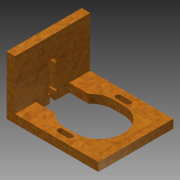
# Autodesk Inventor part: frame_x
Saved by Autodesk Inventor 2014 (Build 180170000, 170)
## iProperties
Created: 2015-01-04
Part Number: frame_x
Material: Generic
Document SubType Name: Modeling
Designer: cruiser
Density: 1 g/cm^3
Appearance: Yellow Pine - Solid Stained Light Low Gloss
Author: cruiser
Autodesk Inventor part; units mm, degrees
ref_plane "YZ Plane" through (0, 0, 0) normal (1, 0, 0) x (0, 1, 0)
ref_plane "XZ Plane" through (0, 0, 0) normal (0, 1, 0) x (-1, 0, 0)
ref_plane "XY Plane" through (0, 0, 0) normal (0, 0, 1) x (1, 0, 0)
sketch "Sketch1" plane through (0, 0, 0) normal (0, 0, 1) x (1, 0, 0)
  circle A0 centre (0, 0) radius 14.5
  circle A1 centre (0, 17.5) radius 1.575
  line L0 (0, 0) -> (14.5, 0)
  circle A2 centre (0, -17.5) radius 1.575
  line L1 (0, 10) -> (-25, 10)
  line L2 (-25, 10) -> (-25, -10)
  line L3 (-25, -10) -> (0, -10)
  line L4 (0, -10) -> (0, 10)
  line L5 (25, -22.5) -> (-25, -22.5)
  line L6 (-25, -22.5) -> (-25, 22.5)
  line L7 (-25, 22.5) -> (25, 22.5)
  line L8 (25, 22.5) -> (25, -22.5)
  line L9 (25, -22.5) -> (-25, 22.5) construction
  line L10 (-25, -22.5) -> (25, 22.5) construction
  dimension "d1" = 29
  dimension "d0" = 3.15
  dimension "d2" = 17.5
  dimension "d3" = 0
  dimension "d4" = 20
  dimension "d5" = 25
  dimension "d6" = 0
  dimension "d7" = 50
  dimension "d8" = 45
  constraints: 22 end point, 4 parallel, 3 horizontal, 2 centre point, 2 midpoint, 2 perpendicular, 1 coincident, 1 horizontal alignment, 1 symmetric about line, 4 other
  measures "d0" diameter of A1
  measures "d2" distance of point (0, 0) A1.centre
  measures "d3" horizontal distance of point (0, 0) A1.centre
  measures "d4" distance of L1.end L2.end
  measures "d5" distance from line of A1.centre L2
  measures "d6" distance from line of L4 point (0, 0)
  measures "d7" distance of L6.end L7.end
  measures "d8" distance of L5.end L6.end
extrude "Extrusion1" add sketch "Sketch1" along normal blind 5.08 contours A0 L1 L6 L7 L8 L5 L3
sketch "Sketch2" plane through (-25, 10, 0) normal (-1, 0, 0) x (0, 0, 1)
  line L0 (0, 0) -> (0, 12.5) projected
  line L1 (0, -32.5) -> (5.08, -32.5)
  line L2 (5.08, -32.5) -> (5.08, 12.5)
  line L3 (5.08, 12.5) -> (0, 12.5)
  line L4 (0, 12.5) -> (0, -32.5)
  line L5 (0, -32.5) -> (5.08, -32.5) projected
  point P0 (0, -10)
  dimension "d11" = 0
  dimension "d12" = 0
  constraints: 8 end point, 2 parallel, 1 horizontal, 1 perpendicular
  measures "d11" distance between parallel lines of L4 L0
  measures "d12" distance between parallel lines of L5 L1
extrude "Extrusion2" add sketch "Sketch2" along normal blind 5.08 separate body
sketch "Sketch3" plane through (-25, -22.5, 5.08) normal (0, 0, 1) x (1, 0, 0)
  line L0 (0, 0) -> (0, 45) projected
  line L1 (0, 45) -> (-5.08, 45) projected
  line L2 (-5.08, 0) -> (-5.08, 45) projected
  line L3 (0, 0) -> (-5.08, 0) projected
  point P0 (25, 22.5)
extrude "Extrusion3" add sketch "Sketch3" along normal blind 30 bodies 2
sketch "Sketch4" plane through (-25, 10, 0) normal (1, 0, 0) x (0, 0, -1)
  line L0 (-35.08, -32.5) -> (-35.08, 12.5) projected
  line L1 (0, 12.5) -> (0, -32.5) projected
  line L2 (-35.08, -10) -> (0, -10)
  arc A0 (-19.58, -8) -> (-22.58, -8) centre (-21.08, -10) ccw
  line L3 (-19.58, -12) -> (-22.58, -12)
  line L4 (-22.58, -12) -> (-22.58, -8)
  line L5 (-22.58, -8) -> (-19.58, -8)
  line L6 (-19.58, -8) -> (-19.58, -12)
  line L7 (-19.58, -12) -> (-22.58, -8) construction
  line L8 (-22.58, -12) -> (-19.58, -8) construction
  line L9 (-5.08, -32.5) -> (-5.08, 12.5) projected
  arc A1 (-18.58, -10) -> (-19.58, -8) centre (-21.08, -10) ccw
  arc A2 (-22.58, -8) -> (-23.58, -10) centre (-21.08, -10) ccw
  arc A3 (-23.58, -10) -> (-22.58, -12) centre (-21.08, -10) ccw
  arc A4 (-22.58, -12) -> (-19.58, -12) centre (-21.08, -10) ccw
  arc A5 (-19.58, -12) -> (-18.58, -10) centre (-21.08, -10) ccw
  line L10 (0, -11.65) -> (-19.58, -11.65)
  line L11 (-19.58, -11.65) -> (-19.58, -8.35)
  line L12 (-19.58, -8.35) -> (0, -8.35)
  line L13 (0, -8.35) -> (0, -11.65)
  line L14 (0, -11.65) -> (-19.58, -8.35) construction
  line L15 (-19.58, -11.65) -> (0, -8.35) construction
  line L16 (-7.5, -12.75) -> (-5, -12.75)
  line L17 (-5, -12.75) -> (-5, -7.25)
  line L18 (-5, -7.25) -> (-7.5, -7.25)
  line L19 (-7.5, -7.25) -> (-7.5, -12.75)
  line L20 (-7.5, -12.75) -> (-5, -7.25) construction
  line L21 (-5, -12.75) -> (-7.5, -7.25) construction
  point P0 (-9.79, -10)
  point P1 (-6.25, -10)
  dimension "d17" = 5
  dimension "d18" = 3
  dimension "d19" = 16
  dimension "d20" = 3.3
  dimension "d21" = 0
  dimension "d22" = 0
  dimension "d23" = 2.5
  dimension "d24" = 5.5
  dimension "d25" = 5
  constraints: 38 end point, 12 point on circle, 7 midpoint, 6 centre point, 6 parallel, 5 point on line, 4 perpendicular, 3 horizontal
  measures "d17" diameter of A0
  measures "d18" distance of L4.end L5.end
  measures "d19" distance from line of L9 A0.centre
  measures "d20" distance of L10.end L11.end
  measures "d21" distance between parallel lines of L1 L13
  measures "d22" distance between parallel lines of L6 L11
  measures "d23" distance of L18.end L17.end
  measures "d24" distance of L17.end L16.end
  measures "d25" distance between parallel lines of L1 L17
extrude "Extrusion4" cut sketch "Sketch4" against normal up to next contours L1 L2 L17 L12 | L1 L10 L17 L2 | L17 L2 L9 L12 | L12 L9 L18 L17 | L17 L10 L9 L2 | L12 L19 L18 L9 | L9 L2 L19 L12 | L17 L16 L9 L10 | L9 L10 L19 L2 | L19 L2 A1 L12 | L9 L16 L19 L10 | L19 L10 A5 L2 | A1 L2 L6 L12 | A5 L10 L6 L2 | L5 A0 | L6 L2 L4 L5 | L6 L3 L4 L2 | A4 L3 bodies 2
sketch "Sketch5" plane through (-25, 10, 0) normal (1, 0, 0) x (0, 0, -1)
  arc A0 (-22.58, -12) -> (-19.58, -12) centre (-21.08, -10) ccw projected
  arc A1 (-19.58, -8) -> (-22.58, -8) centre (-21.08, -10) ccw projected
  line L0 (-13.08, -27.5) -> (-29.08, -27.5)
  line L1 (-29.08, -27.5) -> (-29.08, 7.5)
  line L2 (-29.08, 7.5) -> (-13.08, 7.5)
  line L3 (-13.08, 7.5) -> (-13.08, -27.5)
  line L4 (-13.08, -27.5) -> (-29.08, 7.5) construction
  line L5 (-29.08, -27.5) -> (-13.08, 7.5) construction
  circle A2 centre (-29.08, 7.5) radius 7.5
  circle A3 centre (-29.08, -27.5) radius 7.5
  point P0 (0, -10)
  dimension "d28" = 35
  dimension "d29" = 16
  dimension "d30" = 15
  dimension "d31" = 15
  constraints: 12 end point, 2 centre point, 2 coincident, 2 midpoint, 2 parallel, 1 horizontal, 1 perpendicular
  measures "d28" distance of L0.end L1.end
  measures "d29" diameter of A0.centre L1
  measures "d30" diameter of A2
  measures "d31" diameter of A3
extrude "Extrusion5" [suppressed]
sketch "Sketch6" plane through (0, 0, 0) normal (0, 0, -1) x (-1, 0, 0)
  line L0 (25, 10) -> (30.08, 10)
  line L1 (30.08, 10) -> (30.08, 13)
  line L2 (30.08, 13) -> (25, 13)
  line L3 (25, 13) -> (25, 10)
  line L4 (25, -10) -> (30.08, -10)
  line L5 (30.08, -10) -> (30.08, -13)
  line L6 (30.08, -13) -> (25, -13)
  line L7 (25, -13) -> (25, -10)
  dimension "d34" = 5.08
  dimension "d35" = 3
  dimension "d36" = 3
  constraints: 16 end point, 4 parallel, 2 horizontal, 2 perpendicular, 1 collinear
  measures "d34" distance of L0.start L0.end
  measures "d35" distance of L0.end L1.end
  measures "d36" distance of L4.end L5.end
extrude "Extrusion6" [suppressed]
sketch "Sketch7" plane through (-30.08, 10, 0) normal (-1, 0, 0) x (0, 0, 1)
  line L0 (0, -32.5) -> (35.08, -32.5) projected
  line L1 (0, 12.5) -> (35.08, 12.5) projected
  line L2 (0, 12.5) -> (0, -8.35) projected
  arc A0 (19.58, -12) -> (22.58, -12) centre (21.08, -10) ccw projected
  line L3 (0, -11.65) -> (0, -32.5) projected
  line L4 (0, -20) -> (7.08, -20)
  line L5 (7.08, -20) -> (7.08, -23)
  line L6 (7.08, -23) -> (0, -23)
  line L7 (0, -23) -> (0, -20)
  line L8 (0, -20) -> (5.08, -20) projected
  line L9 (0, 3) -> (7.08, 3)
  line L10 (7.08, 3) -> (7.08, 0)
  line L11 (7.08, 0) -> (0, 0)
  line L12 (0, 0) -> (0, 3)
  line L13 (0, 3) -> (5.08, 3) projected
  line L14 (2.54, 7) -> (4.54, 7) construction
  line L15 (2.54, 5.425) -> (4.54, 5.425)
  line L16 (4.54, 8.575) -> (2.54, 8.575)
  arc A1 (2.54, 8.575) -> (2.54, 5.425) centre (2.54, 7) ccw
  arc A2 (4.54, 5.425) -> (4.54, 8.575) centre (4.54, 7) ccw
  line L17 (21.08, -10) -> (0, -10)
  line L18 (2.54, -27) -> (4.54, -27) construction
  line L19 (2.54, -25.425) -> (4.54, -25.425)
  line L20 (4.54, -28.575) -> (2.54, -28.575)
  arc A3 (2.54, -25.425) -> (2.54, -28.575) centre (2.54, -27) ccw
  arc A4 (4.54, -28.575) -> (4.54, -25.425) centre (4.54, -27) ccw
  point P0 (34.6702, -32.5)
  point P1 (23.4898, 12.5)
  point P2 (3.54, 7)
  point P3 (3.54, -27)
  dimension "d39" = 7.08
  dimension "d40" = 3
  dimension "d41" = 0
  dimension "d42" = 7.08
  dimension "d43" = 3
  dimension "d44" = 0
  dimension "d45" = 3.15
  dimension "d46" = 2.54
  dimension "d47" = 2
  dimension "d61" = 5.5
  constraints: 34 end point, 8 point on circle, 7 symmetric about line, 6 parallel, 4 centre point, 4 tangent, 3 perpendicular, 2 horizontal, 2 point on line, 1 midpoint, 2 other
  measures "d39" distance of L5.end L6.end
  measures "d40" distance of L4.end L5.end
  measures "d41" distance between parallel lines of L4 L8
  measures "d42" distance of L10.end L11.end
  measures "d43" distance of L9.end L10.end
  measures "d44" distance between parallel lines of L13 L9
  measures "d45" diameter of A2
  measures "d46" distance from line of L2 L14.start
  measures "d47" distance of L14.start L14.end
  measures "d61" distance from line of L1 point (3.54, 7)
extrude "Extrusion7" [suppressed]
sketch "Sketch8" plane through (0, 0, 5.08) normal (0, 0, 1) x (1, 0, 0)
  arc A0 (-10.5, -10) -> (-10.5, 10) centre (0, 0) ccw projected
  line L0 (25, -22.5) -> (25, 22.5) projected
  line L1 (25, 22.5) -> (-25, 22.5) projected
  line L2 (-25, 22.5) -> (-25, -22.5) projected
  line L3 (-19.5, 14.25) -> (-22, 14.25)
  line L4 (-22, 14.25) -> (-22, 19.75)
  line L5 (-22, 19.75) -> (-19.5, 19.75)
  line L6 (-19.5, 19.75) -> (-19.5, 14.25)
  line L7 (-19.5, 14.25) -> (-22, 19.75) construction
  line L8 (-22, 14.25) -> (-19.5, 19.75) construction
  line L9 (-15, 15.425) -> (-25, 15.425)
  line L10 (-25, 15.425) -> (-25, 18.575)
  line L11 (-25, 18.575) -> (-15, 18.575)
  line L12 (-15, 18.575) -> (-15, 15.425)
  line L13 (-15, 15.425) -> (-25, 18.575) construction
  line L14 (-25, 15.425) -> (-15, 18.575) construction
  line L15 (0, 0) -> (25, 0)
  line L16 (-19.5, -14.25) -> (-22, -14.25)
  line L17 (-22, -14.25) -> (-22, -19.75)
  line L18 (-22, -19.75) -> (-19.5, -19.75)
  line L19 (-19.5, -19.75) -> (-19.5, -14.25)
  line L20 (-19.5, -14.25) -> (-22, -19.75) construction
  line L21 (-22, -14.25) -> (-19.5, -19.75) construction
  line L22 (-15, -15.425) -> (-25, -15.425)
  line L23 (-25, -15.425) -> (-25, -18.575)
  line L24 (-25, -18.575) -> (-15, -18.575)
  line L25 (-15, -18.575) -> (-15, -15.425)
  line L26 (-15, -15.425) -> (-25, -18.575) construction
  line L27 (-25, -15.425) -> (-15, -18.575) construction
  point P0 (-20, 13)
  point P1 (-20.75, 17)
  point P2 (-20, 17)
  point P3 (-20.75, -17)
  point P4 (-20, -17)
  point P5 (-25, -22.5)
  dimension "d51" = 2.5
  dimension "d52" = 5.5
  dimension "d53" = 3.15
  dimension "d54" = 5.5
  dimension "d55" = 5.5
  dimension "d56" = 3
  dimension "d57" = 0
  dimension "d58" = 10
  constraints: 50 end point, 10 symmetric about line, 9 midpoint, 4 parallel, 2 horizontal, 2 perpendicular, 1 other
  measures "d51" distance of L4.end L5.end
  measures "d52" distance of L3.end L4.end
  measures "d53" distance of L9.end L10.end
  measures "d54" distance from line of point (-20.75, 17) L1
  measures "d55" distance from line of L1 point (-20, 17)
  measures "d57" horizontal extent of L10
  measures "d58" distance of L9.start L9.end
extrude "Extrusion8" [suppressed]
sketch "Sketch9" plane through (0, 0, 0) normal (0, 0, -1) x (-1, 0, 0)
  circle A0 centre (0, 17.5) radius 1.575 projected
  circle A1 centre (0, -17.5) radius 1.575 projected
  arc A2 (10.5, 10) -> (10.5, -10) centre (0, 0) ccw projected
  line L0 (10.5, 10) -> (25, 10) projected
  line L1 (3, 17.5) -> (-3, 17.5) construction
  line L2 (3, 15.925) -> (-3, 15.925)
  line L3 (-3, 19.075) -> (3, 19.075)
  arc A3 (3, 15.925) -> (3, 19.075) centre (3, 17.5) ccw
  arc A4 (-3, 19.075) -> (-3, 15.925) centre (-3, 17.5) ccw
  line L4 (3, -17.5) -> (-3, -17.5) construction
  line L5 (3, -15.925) -> (-3, -15.925)
  line L6 (-3, -19.075) -> (3, -19.075)
  arc A5 (3, -19.075) -> (3, -15.925) centre (3, -17.5) ccw
  arc A6 (-3, -15.925) -> (-3, -19.075) centre (-3, -17.5) ccw
  line L7 (3, 0) -> (-3, 0) construction
  line L8 (3, -14.5) -> (-3, -14.5)
  line L9 (-3, 14.5) -> (3, 14.5)
  arc A7 (3, -14.5) -> (3, 14.5) centre (3, 0) ccw
  arc A8 (-3, 14.5) -> (-3, -14.5) centre (-3, 0) ccw
  dimension "d62" = 3
  dimension "d63" = 0
  dimension "d64" = 3
  dimension "d65" = 0
  dimension "d66" = 3
  dimension "d67" = 0
  constraints: 24 end point, 12 point on circle, 12 tangent, 6 centre point, 6 parallel, 3 midpoint
  measures "d62" distance of A0.centre L1.end
  measures "d63" distance edge to line of A0 L3
  measures "d64" distance of A1.centre L4.end
  measures "d65" distance edge to line of A1 L6
  measures "d66" distance of A2.centre L7.end
  measures "d67" distance edge to line of A2 L8
extrude "Extrusion9" cut sketch "Sketch9" against normal blind 10 contours A0 L3 A3 L2 | A0 L2 A4 L3 | A1 L5 A5 L6 | A1 L6 A6 L5 | L0 A7 L8 A2 | A2 L9 A7 L0 | A2 L8 A8 L9 bodies 1
equation "\"d0\" = m3_diameter"
equation "\"d2\" = 0.5 * stepper_screw_space"
equation "\"d9\" = wood_thickness"
equation "\"d13\" = wood_thickness"
equation "\"d28\" = stepper_screw_space"
equation "\"d34\" = wood_thickness"
equation "\"d37\" = wood_thickness"
equation "\"d45\" = m3_diameter"
equation "\"d46\" = 0.5 * wood_thickness"
equation "\"d49\" = wood_thickness"
equation "\"d59\" = wood_thickness"
equation "\"wood_thickness\" = 5.08"
equation "\"m3_diameter\" = 3.15"
equation "\"m5_diameter\" = 5.25"
equation "\"stepper_screw_space\" = 35"
equation "\"stepper_shaft_diameter\" = 5"
equation "\"stepper_body_diameter\" = 28"
equation "\"laser_body_diameter\" = 12"
body "Solid1"
body "Solid2"
